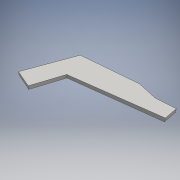
# Autodesk Inventor part: Pivot Link
Saved by Autodesk Inventor 2016 (Build 200138000, 138)
## iProperties
Created: 2016-03-25
Part Number: Pivot Link
Material: Generic
Document SubType Name: Modeling
Designer: Henrik Samuelsson
Density: 1 g/cm^3
Appearance: Default
Author: Henrik Samuelsson
Autodesk Inventor part; units mm, degrees
ref_plane "YZ Plane" through (0, 0, 0) normal (1, 0, 0) x (0, 1, 0)
ref_plane "XZ Plane" through (0, 0, 0) normal (0, 1, 0) x (-1, 0, 0)
ref_plane "XY Plane" through (0, 0, 0) normal (0, 0, 1) x (1, 0, 0)
sketch "Sketch1" plane through (0, 0, 0) normal (0, 0, 1) x (1, 0, 0)
  line L0 (300, 0) -> (300, -90)
  line L1 (300, -90) -> (0, -90)
  line L2 (67.6148, -18.1173) -> (23.6156, -182.3247)
  line L3 (23.6156, -182.3247) -> (-43.9992, -164.2074)
  line L4 (-43.9992, -164.2074) -> (0, 0)
  line L5 (0, 0) -> (67.6148, -18.1173)
  line L6 (0, 0) -> (300, 0)
  line L7 (0, -90) -> (0, 0)
  dimension "d0" = 300
  dimension "d1" = 90
  dimension "d2" = 70
  dimension "d3" = 170
  dimension "d5" = 105
  dimension "d6" = 0
  dimension "d7" = 0
  dimension "d8" = 0
  dimension "d9" = 300
  constraints: 16 end point, 3 perpendicular, 1 horizontal, 1 parallel
  measures "d0" distance of L1.end L0.end
  measures "d1" distance of L0.start L0.end
  measures "d2" distance of L2.end L3.end
  measures "d3" distance of L2.start L2.end
  measures "d5" angle of L6 L4
  measures "d6" distance of point (0, 0) L4.end
  measures "d7" distance of point (0, 0) L4.end
  measures "d8" horizontal distance of point (0, 0) L1.end
  measures "d9" distance of L4.end L0.start
extrude "Extrusion1" add sketch "Sketch1" along normal blind 10
sketch "Sketch2" plane through (0, 0, 10) normal (0, 0, 1) x (1, 0, 0)
  line L0 (300, -90) -> (300, 0) projected
  line L1 (300, -20) -> (300, -60)
  line L2 (23.6156, -182.3247) -> (48.3539, -90) projected
  line L3 (48.3539, -90) -> (300, -60)
  line L4 (300, -20) -> (250, -20)
  line L5 (250, -20) -> (118.443, 27.8828)
  line L6 (48.3539, -90) -> (300, -90) projected
  line L7 (48.3539, -90) -> (300, -90)
  line L8 (300, -90) -> (300, -60)
  line L9 (300, 0) -> (0, 0) projected
  line L10 (195.0505, 0) -> (300, 0)
  line L11 (300, 0) -> (300, -20)
  dimension "d12" = 40
  dimension "d13" = 20
  dimension "d14" = 50
  dimension "d15" = 140
  dimension "d16" = 160
  constraints: 16 end point, 4 point on line, 3 collinear, 1 horizontal, 1 perpendicular
  measures "d12" distance of L1.end L1.start
  measures "d13" distance of L0.end L1.start
  measures "d14" distance of L1.start L4.end
  measures "d15" distance of L4.end L5.end
  measures "d16" angle of L4 L5
extrude "Extrusion2" cut sketch "Sketch2" against normal blind 10
body "Solid1"
